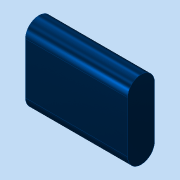
# Autodesk Inventor part: 12V可充电锂电池模型
Saved by Autodesk Inventor 2019 (Build 230136000, 136)
## iProperties
Created: 2020-10-22
Part Number: 12V可充电锂电池模型
Material: 钢，镀锌
Document SubType Name: Modeling
Designer: Wang Hua
Density: 7.85 g/cm^3
Appearance: 镀锌
Author: Wang Hua
Autodesk Inventor part; units mm, degrees
ref_plane "YZ Plane" through (0, 0, 0) normal (1, 0, 0) x (0, 1, 0)
ref_plane "XZ Plane" through (0, 0, 0) normal (0, 1, 0) x (-1, 0, 0)
ref_plane "XY Plane" through (0, 0, 0) normal (0, 0, 1) x (1, 0, 0)
sketch "草图1" plane through (0, 0, 0) normal (0, 0, 1) x (1, 0, 0)
  line L0 (36.22, -27.7) -> (-36.22, -27.7)
  line L1 (-36.22, -27.7) -> (-36.22, 27.7)
  line L2 (-36.22, 27.7) -> (36.22, 27.7)
  line L3 (36.22, 27.7) -> (36.22, -27.7)
  line L4 (36.22, -27.7) -> (-36.22, 27.7) construction
  line L5 (-36.22, -27.7) -> (36.22, 27.7) construction
  point P0 (0, 0)
  dimension "d0" = 55.4
  dimension "d1" = 72.44
  constraints: 12 end point, 2 midpoint, 2 parallel, 1 horizontal, 1 perpendicular
  measures "d0" distance of L2.end L0.start
  measures "d1" distance of L1.end L2.end
extrude "拉伸1" add sketch "草图1" along normal blind 19.1
fillet "圆角1" radius 9.55 4 edges at (0, 27.7, 19.1) (0, 27.7, 0) (0, -27.7, 19.1) (0, -27.7, 0)
